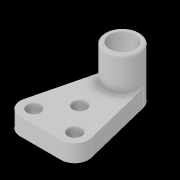
# Autodesk Inventor part: lab9_1
Saved by Autodesk Inventor 2019 (Build 230136000, 136)
## iProperties
Created: 2020-11-25
Part Number: lab9_1
Material: Generic
Document SubType Name: Modeling
Designer: liviu
Density: 1 g/cm^3
Appearance: Default
Author: liviu
Autodesk Inventor part; units mm, degrees
ref_plane "YZ Plane" through (0, 0, 0) normal (1, 0, 0) x (0, 1, 0)
ref_plane "XZ Plane" through (0, 0, 0) normal (0, 1, 0) x (-1, 0, 0)
ref_plane "XY Plane" through (0, 0, 0) normal (0, 0, 1) x (1, 0, 0)
sketch "Sketch1" plane through (0, 0, 0) normal (0, 1, 0) x (-1, 0, 0)
  line L0 (0, 0) -> (12, 0)
  line L1 (19.7639, -9.9292) -> (9.7049, -50.4115)
  line L2 (-9.7049, -50.4115) -> (-19.7639, -9.9292)
  line L3 (-12, 0) -> (0, 0)
  arc A0 (19.7639, -9.9292) -> (12, 0) centre (12, -8) ccw
  arc A1 (-12, 0) -> (-19.7639, -9.9292) centre (-12, -8) ccw
  arc A2 (-9.7049, -50.4115) -> (9.7049, -50.4115) centre (0, -48) ccw
  point P0 (-22.2311, 0)
  dimension "d0" = 8
  dimension "d1" = 24
  dimension "d2" = 10
  dimension "d3" = 40
  constraints: 8 end point, 6 point on circle, 6 tangent, 3 centre point, 3 point on line, 2 equal length, 1 collinear, 1 equal radius, 1 horizontal
  measures "d0" radius of A0
  measures "d1" distance of A1.centre A0.centre
  measures "d2" radius of A2
  measures "d3" vertical distance of A2.centre A1.centre
extrude "Extrusion1" add sketch "Sketch1" along normal blind 10
sketch "Sketch2" plane through (0, 10, 0) normal (0, 1, 0) x (1, 0, 0)
  arc A0 (9.7049, 50.4115) -> (-9.7049, 50.4115) centre (0, 48) ccw projected
  circle A1 centre (0, 48) radius 10
  point P0 (0, 0)
  constraints: 1 coincident, 3 other
extrude "Extrusion2" add sketch "Sketch2" along normal blind 20
sketch "Sketch3" plane through (0, 30, -48) normal (0, 1, 0) x (1, 0, 0)
  arc A0 (-9.7049, 2.4115) -> (9.7049, 2.4115) centre (0, 0) ccw projected
  circle A1 centre (0, 0) radius 7.5
  point P0 (0, -48)
  dimension "d8" = 15
  constraints: 1 centre point, 1 coincident
  measures "d8" diameter of A1
extrude "Extrusion3" cut sketch "Sketch3" against normal through all
sketch "Sketch4" plane through (0, 10, 0) normal (0, 1, 0) x (1, 0, 0)
  arc A0 (-19.7639, 9.9292) -> (-12, 0) centre (-12, 8) ccw projected
  arc A1 (12, 0) -> (19.7639, 9.9292) centre (12, 8) ccw projected
  point P0 (0, 0)
  point P1 (0, 23)
  dimension "d11" = 15
  dimension "d12" = 12
  constraints: 2 coincident
  measures "d11" vertical distance of point (12, 8) point (0, 23)
  measures "d12" horizontal distance of point (12, 8) point (0, 23)
hole "Hole1" at (-12, 10, -8) at (12, 10, -8) at (0, 10, -23) direction (0, -1, 0) diameter 8 end through all
fillet "Fillet1" radius 1 3 edges at (-10, 30, -48) (-1.2147, 10, -38.0741) (9.9259, 10, -49.2147)
body "Solid1"
